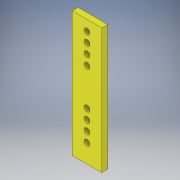
# Autodesk Inventor part: BottomRearLeg
Saved by Autodesk Inventor 2019 (Build 230136000, 136)
## iProperties
Created: 2019-04-01
Part Number: BottomRearLeg
Material: Generic
Document SubType Name: Modeling
Designer: cnam
Density: 1 g/cm^3
Appearance: Default
Author: cnam
Autodesk Inventor part; units mm, degrees
ref_plane "YZ Plane" through (0, 0, 0) normal (1, 0, 0) x (0, 1, 0)
ref_plane "XZ Plane" through (0, 0, 0) normal (0, 1, 0) x (-1, 0, 0)
ref_plane "XY Plane" through (0, 0, 0) normal (0, 0, 1) x (1, 0, 0)
sketch "Sketch1" plane through (0, 0, 0) normal (0, 0, 1) x (1, 0, 0)
  circle A0 centre (0, -30.375) radius 0.875
  line L0 (10, -63.625) -> (10, 47.75)
  line L1 (10, 47.75) -> (-10, 47.75)
  line L2 (-10, 47.75) -> (-10, -63.625)
  line L3 (-10, -63.625) -> (10, -63.625)
  line L4 (6.125, -36.75) -> (6.125, -59.75)
  line L5 (6.125, -59.75) -> (-6.125, -59.75)
  line L6 (-6.125, -59.75) -> (-6.125, -36.75)
  line L7 (-6.125, -36.75) -> (6.125, -36.75)
  circle A1 centre (0, 40.75) radius 2
  circle A2 centre (0, -4.25) radius 2
  circle A3 centre (0, 20.75) radius 2
  circle A4 centre (0, -24.25) radius 2
  circle A5 centre (0, 34.0833) radius 2
  circle A6 centre (0, 27.4167) radius 2
  circle A7 centre (0, -10.9167) radius 2
  circle A8 centre (0, -17.5833) radius 2
  point P0 (0, 0)
  point P1 (0, 0)
  constraints: 16 end point, 9 centre point
extrude "Extrusion1" add sketch "Sketch1" along normal blind 4
sketch "Sketch2" plane through (0, 0, 4) normal (0, 0, 1) x (1, 0, 0)
  line L0 (6.125, -59.75) -> (-6.125, -59.75) projected
  line L1 (-6.125, -59.75) -> (-6.125, -36.75) projected
  line L2 (-6.125, -36.75) -> (6.125, -36.75) projected
  line L3 (6.125, -36.75) -> (6.125, -59.75) projected
  circle A0 centre (0, -17.5833) radius 2 projected
  circle A1 centre (0, -10.9167) radius 2 projected
  circle A2 centre (0, 27.4167) radius 2 projected
  circle A3 centre (0, 34.0833) radius 2 projected
  circle A4 centre (0, -24.25) radius 2 projected
  circle A5 centre (0, 20.75) radius 2 projected
  circle A6 centre (0, -4.25) radius 2 projected
  circle A7 centre (0, 40.75) radius 2 projected
  circle A8 centre (0, -30.375) radius 0.875 projected
  line L4 (10, -63.625) -> (10, 47.75) projected
  line L5 (10, 47.75) -> (-10, 47.75) projected
  line L6 (-10, 47.75) -> (-10, -63.625) projected
  line L7 (-10, -63.625) -> (10, -63.625) projected
  line L8 (-10, -36.75) -> (10, -36.75)
  point P0 (0, 0)
  constraints: 2 end point, 2 point on line, 1 horizontal
extrude "Extrusion2" cut sketch "Sketch2" against normal blind 4 contours L3 L8 L4 L7 L6 L1 L0
sketch "Sketch3" plane through (0, 0, 4) normal (0, 0, 1) x (1, 0, 0)
  line L0 (-10, -36.75) -> (10, -36.75) projected
  line L1 (10, -36.75) -> (10, 47.75) projected
  line L2 (10, 47.75) -> (-10, 47.75) projected
  line L3 (-10, 47.75) -> (-10, -36.75) projected
  circle A0 centre (0, -30.375) radius 0.875 projected
  circle A1 centre (0, 40.75) radius 2 projected
  circle A2 centre (0, -4.25) radius 2 projected
  circle A3 centre (0, 20.75) radius 2 projected
  circle A4 centre (0, -24.25) radius 2 projected
  circle A5 centre (0, 34.0833) radius 2 projected
  circle A6 centre (0, 27.4167) radius 2 projected
  circle A7 centre (0, -10.9167) radius 2 projected
  circle A8 centre (0, -17.5833) radius 2 projected
  point P0 (0, 0)
extrude "Extrusion3" add sketch "Sketch3" against normal blind 4 contours A0
sketch "Sketch4" plane through (0, 0, 4) normal (0, 0, 1) x (1, 0, 0)
  line L0 (-10, -36.75) -> (10, -36.75) projected
  line L1 (10, -36.75) -> (10, 47.75) projected
  line L2 (10, 47.75) -> (-10, 47.75) projected
  line L3 (-10, 47.75) -> (-10, -36.75) projected
  circle A0 centre (0, 40.75) radius 2 projected
  circle A1 centre (0, -4.25) radius 2 projected
  circle A2 centre (0, 20.75) radius 2 projected
  circle A3 centre (0, -24.25) radius 2 projected
  circle A4 centre (0, 34.0833) radius 2 projected
  circle A5 centre (0, 27.4167) radius 2 projected
  circle A6 centre (0, -10.9167) radius 2 projected
  circle A7 centre (0, -17.5833) radius 2 projected
  line L4 (-33.7924, 18.25) -> (39.8102, 18.25) construction
  point P0 (0, 0)
  dimension "d6" = 22.5
  constraints: 2 end point, 1 horizontal
  measures "d6" distance from line of L4 A0.centre
body "Solid1"
